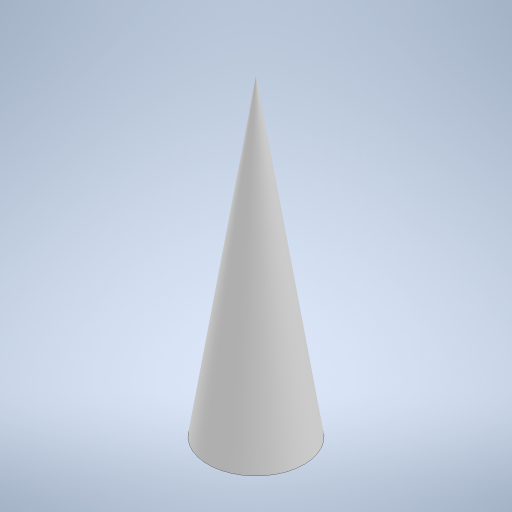
# Autodesk Inventor part: Tip
Saved by Autodesk Inventor 2024.2 (Build 282272000, 272)
## iProperties
Created: 2024-03-06
Part Number: Tip
Material: Generic
Document SubType Name: Modeling
Designer: parmo
Density: 1 g/cm^3
Appearance: Default
Author: parmo
Autodesk Inventor part; units mm, degrees
ref_plane "YZ Plane" through (0, 0, 0) normal (1, 0, 0) x (0, 1, 0)
ref_plane "XZ Plane" through (0, 0, 0) normal (0, 1, 0) x (-1, 0, 0)
ref_plane "XY Plane" through (0, 0, 0) normal (0, 0, 1) x (1, 0, 0)
sketch "Sketch1" plane through (0, 0, 0) normal (0, 0, 1) x (1, 0, 0)
  line L0 (0, 0) -> (0, 39)
  line L1 (0, 0) -> (6, 0)
  line L2 (6, 0) -> (0, 39)
  dimension "d1" = 39
  dimension "d2" = 6
  constraints: 6 end point, 1 horizontal, 1 vertical
  measures "d1" distance of L0.start L0.end
  measures "d2" distance of L0.start L1.end
revolve "Revolution1" add sketch "Sketch1" angle 360 about axis through (0, 0, 0) along (0, 1, 0)
body "Solid1"
